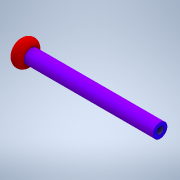
# Autodesk Inventor part: handle
Saved by Autodesk Inventor 2021 (Build 250183000, 183)
## iProperties
Created: 2021-07-29
Part Number: handle
Material: Generic
Document SubType Name: Modeling
Designer: Shammy Haider
Density: 1 g/cm^3
Appearance: Default
Author: Shammy Haider
Autodesk Inventor part; units mm, degrees
ref_plane "YZ Plane" through (0, 0, 0) normal (1, 0, 0) x (0, 1, 0)
ref_plane "XZ Plane" through (0, 0, 0) normal (0, 1, 0) x (-1, 0, 0)
ref_plane "XY Plane" through (0, 0, 0) normal (0, 0, 1) x (1, 0, 0)
sketch "Sketch1" plane through (0, 0, 0) normal (0, 0, 1) x (1, 0, 0)
  line L0 (0, 0) -> (100, 0)
  line L1 (8, 5) -> (100, 5)
  arc A0 (8, 5) -> (0, 5) centre (4, 5) ccw
  line L2 (100, 5) -> (100, 2.38)
  line L3 (100, 2.38) -> (88, 2.38)
  line L4 (88, 2.38) -> (86.6259, 0)
  line L5 (86.6259, 0) -> (0, 0)
  line L6 (0, 5) -> (0, 0)
  dimension "d0" = 100
  dimension "d1" = 5
  dimension "d2" = 92
  dimension "d3" = 4
  dimension "d4" = 12
  dimension "d5" = 120
  dimension "d6" = 2.38
  constraints: 14 end point, 2 horizontal, 2 perpendicular, 2 point on circle, 1 centre point, 1 collinear, 1 point on line, 1 vertical, 1 vertical alignment
  measures "d0" distance of L0.start L0.end
  measures "d1" distance between parallel lines of L0 L1
  measures "d2" distance of L1.start L1.end
  measures "d3" radius of A0
  measures "d4" distance of L2.end L3.end
  measures "d5" angle of L4 L3
  measures "d6" distance from line of L0.end L3
revolve "Revolution1" add sketch "Sketch1" angle 360 about axis through (0, 0, 0) along (1, 0, 0)
thread "Thread1" size "M5x0.8" class "6H" standard "ANSI Metric M Profile" full length
body "Solid1"
